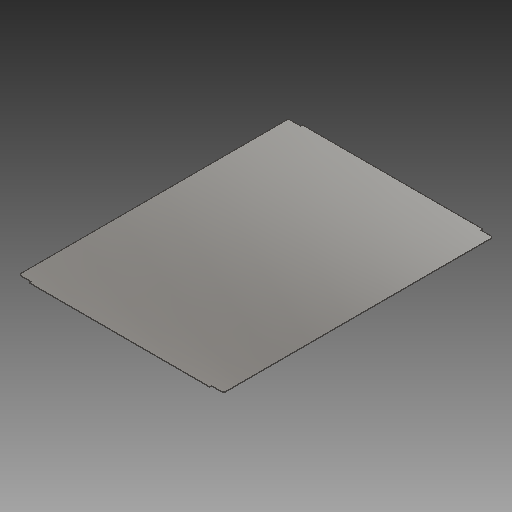
# Autodesk Inventor part: BrennerHalter
Saved by Autodesk Inventor 2018 (Build 220112000, 112)
## iProperties
Created: 2017-10-08
Part Number: BrennerHalter
Material: Edelstahl
Document SubType Name: Blech
Designer: jro
Density: 8 g/cm^3
Sheet Metal Rule: Standard
Appearance: Halbpoliert
toleranz: 1,000 mm
Author: jro
Autodesk Inventor part; units mm, degrees
ref_plane "YZ Plane" through (0, 0, 0) normal (1, 0, 0) x (0, 1, 0)
ref_plane "XZ Plane" through (0, 0, 0) normal (0, 1, 0) x (-1, 0, 0)
ref_plane "XY Plane" through (0, 0, 0) normal (0, 0, 1) x (1, 0, 0)
sketch "Skizze1" plane through (0, 0, 0) normal (0, 0, 1) x (1, 0, 0)
  line L0 (0, 2) -> (-143, 2)
  line L1 (25.4999, 293) -> (34.9999, 293)
  line L2 (-177.9999, 293) -> (-168.4999, 293)
  line L3 (38.4999, 289.9629) -> (38.4999, 7.0371)
  line L4 (-181.4999, 7.0371) -> (-181.4999, 289.9629)
  line L5 (35.13, 4) -> (25.4999, 4)
  line L6 (-178.13, 4) -> (-168.4999, 4)
  spline S0 degree 3 poles (36.4999, 4) (36.9764, 4) (37.5632, 4.2103) (37.9584, 4.6315) (38.3246, 5.0217) (38.4999, 5.5585) (38.4999, 6) knots 2.540569 2.540569 2.540569 2.540569 3.164504 3.164504 3.164504 3.742616 3.742616 3.742616 3.742616
  line L7 (35.13, 4) -> (36.4999, 4)
  line L8 (38.4999, 6) -> (38.4999, 7.0371)
  line L9 (25.4999, 4) -> (25.4999, 2)
  line L10 (35.4629, 2) -> (10, 2)
  line L11 (10, 0) -> (10, 2)
  line L12 (0, 0) -> (10, 0)
  line L13 (10, 2) -> (0, 2)
  line L14 (-143, 0) -> (0, 0)
  line L15 (-153, 0) -> (-143, 0)
  line L16 (-143, 2) -> (-153, 2)
  line L17 (-153, 0) -> (-153, 2)
  line L18 (-153, 2) -> (-178.4629, 2)
  line L19 (-168.4999, 4) -> (-168.4999, 2)
  line L20 (-178.13, 4) -> (-168.4999, 4)
  spline S1 degree 3 poles (38.4999, 291) (38.4999, 291.4765) (38.2896, 292.0633) (37.8684, 292.4585) (37.4782, 292.8247) (36.9414, 293) (36.4999, 293) knots 2.540569 2.540569 2.540569 2.540569 3.164504 3.164504 3.164504 3.742616 3.742616 3.742616 3.742616
  arc A0 (35.13, 291.5858) -> (36.4999, 289.9629) centre (38.7619, 293.2619) ccw
  spline S2 degree 3 poles (38.4999, 289.9629) (38.4999, 289.4925) (38.2896, 289.2439) (37.8684, 289.263) (37.4782, 289.2807) (36.9414, 289.527) (36.4999, 289.9629) knots 0.969773 0.969773 0.969773 0.969773 1.593708 1.593708 1.593708 2.17182 2.17182 2.17182 2.17182
  line L21 (38.4999, 289.9629) -> (38.4999, 291)
  spline S3 degree 3 poles (36.4999, 293) (36.9764, 293) (37.5632, 292.7897) (37.9584, 292.3685) (38.3246, 291.9783) (38.4999, 291.4415) (38.4999, 291) knots -0.601023 -0.601023 -0.601023 -0.601023 0.022912 0.022912 0.022912 0.601023 0.601023 0.601023 0.601023
  spline S4 degree 3 poles (36.4999, 293) (36.9764, 293) (37.5632, 292.7897) (37.9584, 292.3685) (38.3246, 291.9783) (38.4999, 291.4415) (38.4999, 291) knots -0.601023 -0.601023 -0.601023 -0.601023 0.022912 0.022912 0.022912 0.601023 0.601023 0.601023 0.601023
  line L22 (36.4999, 293) -> (35.13, 293)
  line L23 (-175.4999, 295) -> (32.4999, 295)
  line L24 (25.4999, 295) -> (25.4999, 293)
  line L25 (-168.4999, 293) -> (-168.4999, 295)
  line L26 (-178.13, 293) -> (-179.4999, 293)
  spline S5 degree 3 poles (-179.4999, 293) (-179.9764, 293) (-180.5632, 292.7897) (-180.9584, 292.3685) (-181.3246, 291.9783) (-181.4999, 291.4415) (-181.4999, 291) knots -0.601023 -0.601023 -0.601023 -0.601023 0.022912 0.022912 0.022912 0.601023 0.601023 0.601023 0.601023
  line L27 (-181.4999, 291) -> (-181.4999, 289.9629)
  spline S6 degree 3 poles (-181.4999, 289.9629) (-181.4999, 289.4925) (-181.2896, 289.2439) (-180.8684, 289.263) (-180.4782, 289.2807) (-179.9414, 289.527) (-179.4999, 289.9629) knots 0.969773 0.969773 0.969773 0.969773 1.593708 1.593708 1.593708 2.17182 2.17182 2.17182 2.17182
  line L28 (-178.13, 293) -> (-179.4999, 293)
  line L29 (-178.13, 295) -> (-178.13, 293)
  line L30 (-177.9999, 293) -> (-168.4999, 293)
  line L31 (-178.13, 293) -> (-177.9999, 293)
  line L32 (35.13, 293) -> (34.9999, 293)
  line L33 (36.4999, 293) -> (35.13, 293)
  line L34 (25.4999, 293) -> (34.9999, 293)
  line L35 (37.4999, 7) -> (37.4999, 290)
  line L36 (-180.4999, 290) -> (-180.4999, 7)
  line L37 (24.4999, 294) -> (24.4999, 292)
  line L38 (24.4999, 292) -> (35.4999, 292)
  line L39 (37.4999, 292) -> (37.4999, 294.7)
  arc A1 (37.4999, 290) -> (35.4999, 292) centre (35.4999, 290) ccw
  line L40 (-167.4999, 294) -> (-167.4999, 292)
  line L41 (-167.4999, 292) -> (-178.4999, 292)
  line L42 (-180.4999, 292) -> (-180.4999, 294.7)
  arc A2 (-178.4999, 292) -> (-180.4999, 290) centre (-178.4999, 290) ccw
  spline S7 degree 3 poles (-179.4999, 7.0371) (-179.9764, 7.5075) (-180.5632, 7.7561) (-180.9584, 7.737) (-181.3246, 7.7193) (-181.4999, 7.473) (-181.4999, 7.0371) knots -2.17182 -2.17182 -2.17182 -2.17182 -1.547885 -1.547885 -1.547885 -0.969773 -0.969773 -0.969773 -0.969773
  line L43 (-181.4999, 7.0371) -> (-181.4999, 6)
  spline S8 degree 3 poles (-181.4999, 6) (-181.4999, 5.5235) (-181.2896, 4.9367) (-180.8684, 4.5415) (-180.4782, 4.1753) (-179.9414, 4) (-179.4999, 4) knots -0.601023 -0.601023 -0.601023 -0.601023 0.022912 0.022912 0.022912 0.601023 0.601023 0.601023 0.601023
  line L44 (-179.4999, 4) -> (-178.13, 4)
  line L45 (-178.13, 4) -> (-168.4999, 4)
  spline S9 degree 3 poles (38.4999, 7.0371) (38.4999, 7.5075) (38.2896, 7.7561) (37.8684, 7.737) (37.4782, 7.7193) (36.9414, 7.473) (36.4999, 7.0371) knots -2.17182 -2.17182 -2.17182 -2.17182 -1.547885 -1.547885 -1.547885 -0.969773 -0.969773 -0.969773 -0.969773
  line L46 (38.4999, 6) -> (38.4999, 7.0371)
  spline S10 degree 3 poles (36.4999, 4) (36.9764, 4) (37.5632, 4.2103) (37.9584, 4.6315) (38.3246, 5.0217) (38.4999, 5.5585) (38.4999, 6) knots 2.540569 2.540569 2.540569 2.540569 3.164504 3.164504 3.164504 3.742616 3.742616 3.742616 3.742616
  line L47 (35.13, 4) -> (36.4999, 4)
  line L48 (24.4999, 3) -> (24.4999, 5)
  line L49 (24.4999, 5) -> (35.4999, 5)
  line L50 (37.4999, 5) -> (37.4999, 2.3)
  line L51 (-167.4999, 3) -> (-167.4999, 5)
  line L52 (-167.4999, 5) -> (-178.4999, 5)
  line L53 (-180.4999, 5) -> (-180.4999, 2.3)
  arc A3 (-180.4999, 7) -> (-178.4999, 5) centre (-178.4999, 7) ccw
  arc A4 (35.4999, 5) -> (37.4999, 7) centre (35.4999, 7) ccw
  line L54 (-180.4999, 2.3) -> (-178.13, 2.3)
  spline S11 degree 3 poles (-179.4999, 7.0371) (-179.9764, 7.5075) (-180.5632, 7.7561) (-180.9584, 7.737) (-181.3246, 7.7193) (-181.4999, 7.473) (-181.4999, 7.0371) knots -2.17182 -2.17182 -2.17182 -2.17182 -1.547885 -1.547885 -1.547885 -0.969773 -0.969773 -0.969773 -0.969773
  spline S12 degree 3 poles (-179.4999, 7.0371) (-179.9764, 7.5075) (-180.5632, 7.7561) (-180.9584, 7.737) (-181.3246, 7.7193) (-181.4999, 7.473) (-181.4999, 7.0371) knots -2.17182 -2.17182 -2.17182 -2.17182 -1.547885 -1.547885 -1.547885 -0.969773 -0.969773 -0.969773 -0.969773
  spline S13 degree 3 poles (-179.4999, 7.0371) (-179.9764, 7.5075) (-180.5632, 7.7561) (-180.9584, 7.737) (-181.3246, 7.7193) (-181.4999, 7.473) (-181.4999, 7.0371) knots -2.17182 -2.17182 -2.17182 -2.17182 -1.547885 -1.547885 -1.547885 -0.969773 -0.969773 -0.969773 -0.969773
  line L55 (24.4999, 3) -> (-167.4999, 3)
  line L56 (24.4999, 294) -> (-167.4999, 294)
  dimension "toleranz" = 1
  dimension "d1" = 1
  dimension "d5" = 1
  dimension "d6" = 1
  dimension "eckenradius" = 2
  dimension "d8" = 1
  dimension "d9" = 1
  dimension "d10" = 2
  dimension "d11" = 1
  dimension "d12" = 1
  dimension "d13" = 1
  dimension "d14" = 1
  dimension "d16" = 2
  dimension "d17" = 1
  dimension "d18" = 1
  measures "toleranz" distance between parallel lines of L3 L35
  measures "d1" distance between parallel lines of L4 L36
  measures "d5" distance between parallel lines of L37 L24
  measures "d6" distance between parallel lines of L38 L1
  measures "eckenradius" radius of A1
  measures "d8" distance between parallel lines of L2 L41
  measures "d9" distance between parallel lines of L25 L40
  measures "d10" radius of A2
  measures "d11" distance between parallel lines of L5 L49
  measures "d12" distance between parallel lines of L9 L48
  measures "d13" distance between parallel lines of L19 L51
  measures "d14" distance between parallel lines of L45 L52
  measures "d16" radius of A3
  measures "d17" distance between parallel lines of L10 L55
  measures "d18" distance between parallel lines of L56 L23
extrude "Grobblech2" add sketch "Skizze1" along normal blind 0.5 contours L35 A4 L49 L48 L55 L51 L52 A3 L36 A2 L41 L40 L56 L37 L38 A1
equation "\"d1\" = toleranz"
equation "\"d5\" = toleranz"
equation "\"d6\" = toleranz"
equation "\"d8\" = toleranz"
equation "\"d9\" = toleranz"
equation "\"d10\" = eckenradius"
equation "\"d11\" = toleranz"
equation "\"d12\" = toleranz"
equation "\"d13\" = toleranz"
equation "\"d14\" = toleranz"
equation "\"d16\" = eckenradius"
equation "\"d17\" = toleranz"
equation "\"d18\" = toleranz"
equation "\"d19\" = Stärke"
equation "\"d3\" = toleranz"
equation "\"Biegeradius\" = Stärke"
equation "\"BreiteBiegungsfreistellung\" = Stärke"
equation "\"TiefeBiegungsfreistellung\" = 0.5 * Stärke"
equation "\"GrößeEckenfreistellung\" = 4 * Stärke"
equation "\"MinimalRest\" = 2 * Stärke"
equation "\"Übergangsradius\" = Biegeradius"
equation "\"JacobiRadiusGröße\" = Stärke"
equation "\"Abstandsgröße\" = Stärke"
equation "\"Stärke\" = 0.5"
